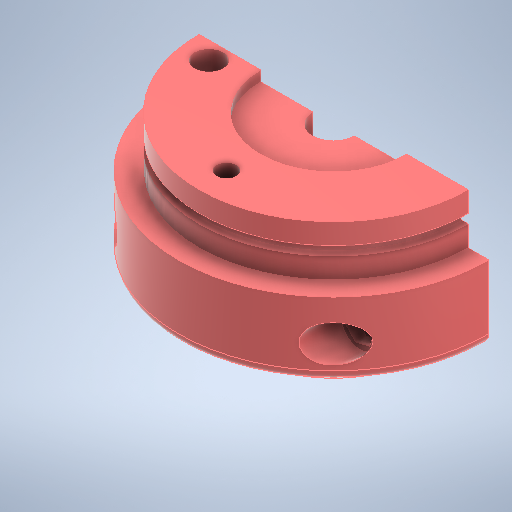
# Autodesk Inventor part: cap3_v0.7.0
Saved by Autodesk Inventor 2025 (Build 290162000, 162)
## iProperties
Created: 2026-01-12
Part Number: cap3_v0.7.0
Material: ABS Plastic
Document SubType Name: Modeling
Designer: SLM30
Density: 1.06 g/cm^3
Appearance: Smooth - Red
Author: SLM30
Autodesk Inventor part; units mm, degrees
ref_plane "YZ Plane" through (0, 0, 0) normal (1, 0, 0) x (0, 1, 0)
ref_plane "XZ Plane" through (0, 0, 0) normal (0, 1, 0) x (-1, 0, 0)
sketch "Sketch1" plane through (0, 0, 0) normal (0, 0, 1) x (1, 0, 0)
  line L0 (0, 0) -> (-14, 0)
  line L1 (-14, 0) -> (-14, 2)
  line L2 (-14, 2) -> (-25.825, 2)
  line L3 (-25.825, 2) -> (-25.825, -7.7)
  line L4 (-25.825, -7.7) -> (-29.825, -7.7)
  line L5 (0, 0) -> (0, -10)
  line L6 (0, -10) -> (-16, -10)
  line L7 (-16, -10) -> (-16, -21)
  line L8 (-16, -21) -> (0, -21)
  line L9 (0, -21) -> (0, -31)
  line L10 (0, -31) -> (-16, -31)
  line L11 (-29.825, -7.7) -> (-29.825, -21)
  line L12 (-29.825, -21) -> (-16, -31)
  arc A0 (-24.6268, -3.7009) -> (-24.6268, -2.0009) centre (-25.325, -2.8509) ccw
  line L13 (-25.825, -2.0009) -> (-24.6268, -2.0009)
  line L14 (-25.825, -3.7009) -> (-24.6268, -3.7009)
  line L15 (0, -37.6) -> (0, 8.6) projected
  dimension "d0" = 14
  dimension "d1" = 2
  dimension "d2" = 11.825
  dimension "d3" = 9.7
  dimension "d4" = 4
  dimension "d5" = 10
  dimension "d6" = 16
  dimension "d7" = 11
  dimension "d8" = 10
  dimension "d9" = 13.825
  dimension "d10" = 125.879
  dimension "d11" = 1.7
  dimension "d12" = 1.1
  dimension "d13" = 0.5
  dimension "d14" = 0.85
  dimension "d15" = 4.0009
  constraints: 30 end point, 7 perpendicular, 4 point on line, 3 horizontal, 2 point on circle, 2 vertical, 1 centre point, 1 parallel
  measures "d0" distance of L0.start L0.end
  measures "d1" distance of L0.end L1.end
  measures "d2" distance of L1.end L2.end
  measures "d3" distance of L2.end L3.end
  measures "d4" distance of L3.end L4.end
  measures "d5" distance of L0.start L5.end
  measures "d6" distance of L5.end L6.end
  measures "d7" distance of L6.end L7.end
  measures "d8" distance of L8.end L9.end
  measures "d9" horizontal distance of L11.end L10.end
  measures "d10" angle of L11 L12
  measures "d11" distance of L14.start L13.start
  measures "d12" radius of A0
  measures "d13" distance from line of L3 A0.centre
  measures "d14" distance from line of L14 A0.centre
  measures "d15" distance between parallel lines of L2 L13
revolve "Revolution1" add sketch "Sketch1" angle 180 about axis through (0, -10, 0) along (0, 1, 0) contours L5 L6 L7 L8 L9 L10 L12 L11 L4 L3 L14 A0 L13 L2 L1 L0
sketch "Sketch2" plane through (16, -31, 0) normal (0, 0, -1) x (-1, 0, 0)
  circle A0 centre (5, 15.5) radius 2.25
  line L0 (0, 10) -> (0, 21) projected
  line L1 (32, 21) -> (0, 21) projected
  point P0 (16, 31)
  dimension "d17" = 4.5
  dimension "d18" = 5
  dimension "d19" = 5.5
  constraints: 1 centre point
  measures "d17" diameter of A0
  measures "d18" distance from line of L0 A0.centre
  measures "d19" distance from line of L1 A0.centre
hole "Hole1" at (11, -15.5, 0) direction (0, 0, 1) diameter 4.5 depth 21.25
mirror "Mirror1" about plane through (0, 0, 0) normal (1, 0, 0) of "Hole1"
sketch "Sketch3" plane through (0, 0, 0) normal (0, 1, 0) x (1, 0, 0)
  circle A0 centre (0, 0) radius 4
  dimension "d27" = 8
  constraints: 1 centre point, 1 coincident
  measures "d27" diameter of A0
hole "Hole2" at (0, 0, 0) direction (0, -1, 0) diameter 8 depth 10
sketch "Sketch4" plane through (-16, -31, 0) normal (0, -1, 0) x (1, 0, 0)
  circle A0 centre (16, 0) radius 7
  dimension "d35" = 14
  constraints: 1 centre point, 1 coincident
  measures "d35" diameter of A0
hole "Hole3" at (0, -31, 0) direction (0, 1, 0) diameter 14 depth 10
sketch "Sketch5" plane through (-25.825, 2, 0) normal (0, 1, 0) x (1, 0, 0)
  circle A0 centre (5.224, -3.354) radius 2.75
  circle A1 centre (25.225, -20.001) radius 1.9085
  point P0 (25.825, 0)
  dimension "d43" = 5.5
  dimension "d44" = 3.817
  dimension "d45" = 20.601
  dimension "d46" = 20.001
  dimension "d47" = 16.647
  dimension "d48" = 20.001
  constraints: 2 centre point
  measures "d43" diameter of A0
  measures "d44" diameter of A1
  measures "d45" horizontal distance of point (25.825, 0) A0.centre
  measures "d46" vertical distance of point (25.825, 0) A1.centre
  measures "d47" vertical distance of A1.centre A0.centre
  measures "d48" horizontal distance of A0.centre A1.centre
sketch "Sketch6" plane through (-25.825, 2, 0) normal (0, 1, 0) x (1, 0, 0)
  circle A0 centre (25.225, -20.001) radius 1.9085
  line L0 (29.825, 0) -> (39.825, 0) projected
  circle A1 centre (5.224, -3.354) radius 2.75
  point P0 (25.825, 0)
  dimension "d49" = 3.817
  dimension "d50" = 20.001
  dimension "d51" = 5.5
  dimension "d52" = 20.601
  dimension "d53" = 16.647
  dimension "d54" = 20.001
  constraints: 2 centre point
  measures "d49" diameter of A0
  measures "d50" distance from line of L0 A0.centre
  measures "d51" diameter of A1
  measures "d52" horizontal distance of point (25.825, 0) A1.centre
  measures "d53" vertical distance of A0.centre A1.centre
  measures "d54" horizontal distance of A1.centre A0.centre
hole "Hole4" at (-0.6, 2, 20.001) direction (0, -1, 0) diameter 3.817 end through all
hole "Hole5" at (-20.601, 2, 3.354) direction (0, -1, 0) diameter 5.5 depth 5
sketch "Sketch7" plane through (0, -31, 0) normal (0, -1, 0) x (1, 0, 0)
  circle A0 centre (-0.6, 20.001) radius 1.9085 projected
  circle A1 centre (-0.6, 20.001) radius 3.5
  point P0 (0, 0)
  dimension "d69" = 7
  constraints: 1 centre point, 1 coincident
  measures "d69" diameter of A1
hole "Hole6" at (-0.6, -31, 20.001) direction (0, 1, 0) diameter 7 depth 7
ref_plane "Work Plane1" through (0, 0, 30) normal (0, 0, 1) x (1, 0, 0)
sketch "Sketch8" plane through (25.825, 2, 0) normal (0, 0, -1) x (-1, 0, 0)
  circle A0 centre (4.825, -17.5) radius 1.75
  line L0 (55.65, -23) -> (-4, -23) projected
  line L1 (9.825, -23) -> (9.825, -12) projected
  point P0 (25.825, -2)
  dimension "d78" = 3.5
  dimension "d79" = 5.5
  dimension "d80" = 5
  constraints: 1 centre point
  measures "d78" diameter of A0
  measures "d79" distance from line of A0.centre L0
  measures "d80" distance from line of L1 A0.centre
hole "Hole7" at (21, -15.5, 0) direction (0, 0, 1) diameter 3.5 end through all
mirror "Mirror2" about plane through (0, 0, 0) normal (1, 0, 0) of "Hole7"
sketch "Sketch9" plane through (0, 0, 30) normal (0, 0, 1) x (1, 0, 0)
  circle A0 centre (-21, -15.5) radius 1.75 projected
  circle A1 centre (-21, -15.5) radius 3.5
  point P0 (0, 0)
  dimension "d88" = 7
  constraints: 1 centre point, 1 coincident
  measures "d88" diameter of A1
hole "Hole8" at (-21, -15.5, 30) direction (0, 0, -1) diameter 7 depth 14
mirror "Mirror3" about plane through (0, 0, 0) normal (1, 0, 0) of "Hole8"
sketch "Sketch10" plane through (0, 0, 30) normal (0, 0, 1) x (1, 0, 0)
  circle A0 centre (-21, -15.5) radius 1.75 projected
  line L0 (-20.2314, -18.15) -> (-22.9106, -17.4907)
  line L1 (-22.9106, -17.4907) -> (-23.6793, -14.8407)
  line L2 (-23.6793, -14.8407) -> (-21.7686, -12.85)
  line L3 (-21.7686, -12.85) -> (-19.0894, -13.5093)
  line L4 (-19.0894, -13.5093) -> (-18.3207, -16.1593)
  line L5 (-18.3207, -16.1593) -> (-20.2314, -18.15)
  point P0 (0, 0)
  dimension "d96" = 2.65
  constraints: 12 end point, 1 coincident, 13 other
  measures "d96" vertical distance of L0.start point (-21, -15.5)
extrude "Extrusion1" cut sketch "Sketch10" against normal blind 16
mirror "Mirror4" about plane through (0, 0, 0) normal (1, 0, 0) of "Extrusion1"
fillet "Fillet1" radius 2 1 edges at (0, -21, 29.825)
body "Solid1"
